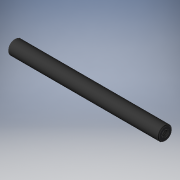
# Autodesk Inventor part: RDOB8-86-WMC4
Saved by Autodesk Inventor 2019 (Build 230136000, 136)
## iProperties
Created: 2022-12-28
Part Number: RDOB8-86-WMC4
Material: Generic
Catalog Web Link: www.cadenas.de
Description: RDOC, RDOB, RDOM, RDSS, RDSSB, RDSSM, RD435S-Rods - Material 1045 Carbon Steel, 1018 Carbon Steel, 4137 Alloy Steel - Outer Diameter Selectable Type
Vendor: MISUMI
Document SubType Name: Modeling
Designer: psAdmin
Manufacturer: MISUMI
Mass: 4.16076 g
Surface Area: 24.2921 cm^2
Volume: 4.16076 cm^3
Density: 1 g/cm^3
Appearance: PSOLRGB-175-175-175
Category: PARTsolutions
Company: MISUMI
Title: RDOB8-86-WMC4
Author: Cadenas PARTsolutions
Comments: Rods - Material 1045 Carbon Steel, 1018 Carbon Steel, 4137 Alloy Steel - Outer Diameter Selectable Type
PSOL_IDENT_0: {$CADENAS_DATA/23d-libs/misumi/metric/22_rods_pipes/rdoc.prj},232 {VTYP=3D},{NB=RDOB8-86-WMC4},{LINA=
PSOL_IDENT_1: RDOB8-86-WMC4},{NN=RDOC, RDOB, RDOM, RDSS, RDSSB, RDSSM, RD435S},{DATE=07.06.2021 02:47:19},{GEOMDAT
PSOL_IDENT_2: E=07.10.2015 00:00:37},{VERSION=},{LINEID=50},{WBVAR=MAT,ST,L,ALT1,MC,WMC},{WBNUMERIC=L,MC,WMC}  {NB=
PSOL_IDENT_3: RDOB8-86-WMC4},{LINA=RDOB8-86-WMC4},{KT=DUMMY},{PN=RDOB8-86-WMC4},{TYPE=RDOB},{MAT=1},{ST=2},{STA='1'
PSOL_IDENT_4: ,'-','2','Black Oxide','3','Electroless Nickel Plating'},{D=8},{DTOL=0/-0.1},{L=86},{LTOL=+/-0.3},{L
PSOL_IDENT_5: 1=[10:500/1]},{C=0.5},{ALT1=2},{ALT1A='3','w/o Tapping','1','with MC (One End Tapping)','2','with WM
PSOL_IDENT_6: C (Both Ends Tapping)'},{MC=0},{MCSA=0},{MCS1=3,4},{WMC=4},{WMCSA=3,4},{WMCS1=3,4},{MMAX=4},{P=0.70}
PSOL_IDENT_7: ,{KDM=3.242},{MATA= '1', '1045 Carbon Steel Equivalent', '2', '1018 Carbon Steel' , '3' , 'SCM435' }
NB: RDOB8-86-WMC4
NN: RDOC, RDOB, RDOM, RDSS, RDSSB, RDSSM, RD435S
NT: Rods - Material 1045 Carbon Steel, 1018 Carbon Steel, 4137 Alloy Steel - Outer Diameter Selectable Type
NBSYN: $PN.
LINA: RDOB8-86-WMC4
CATALOG: Misumi
PN: RDOB8-86-WMC4
MAT: 1045 Carbon Steel Equivalent
ST: Black Oxide
D: 8
DTOL: 0/-0.1
L: 86
LTOL: +/-0.3
C: 0.5
ALT1: with WMC (Both Ends Tapping)
MC: 0
WMC: 4
SUPPLIER: MISUMI
ARTICLENO: RDOB8-86-WMC4
BOMINFO: RDOB8-86-WMC4
CREATOR: CADENAS GmbH
Autodesk Inventor part; units mm, degrees
ref_plane "YZ Plane" through (0, 0, 0) normal (1, 0, 0) x (0, 1, 0)
ref_plane "XZ Plane" through (0, 0, 0) normal (0, 1, 0) x (-1, 0, 0)
ref_plane "XY Plane" through (0, 0, 0) normal (0, 0, 1) x (1, 0, 0)
sketch "Sketch_1" plane through (0, 0, 0) normal (0, 0, 1) x (1, 0, 0)
  line L0 (86, 0) -> (0, 0)
  line L1 (0, 0) -> (0, 3.5)
  line L2 (0, 3.5) -> (0.5, 4)
  line L3 (0.5, 4) -> (85.5, 4)
  line L4 (85.5, 4) -> (86, 3.5)
  line L5 (86, 3.5) -> (86, 0)
  line L6 (86, 0) -> (0, 0)
  constraints: 14 end point
revolve "Revolution1" add sketch "Sketch_1" angle 360 about axis through (86, 0, 0) along (1, 0, 0)
sketch "Sketch2" plane through (0, 0, 0) normal (-1, 0, 0) x (0, 0, 1)
  point P0 (0, 0)
hole "Hole1" at (0, 0, 0) direction (1, 0, 0) diameter 3.242 depth 9.0641 tip angle 120 countersink diameter 4 countersink angle 90 thread size "M4x0.7" class "6H" standard "ISO Metric profile"
sketch "Sketch3" plane through (86, 0, 0) normal (1, 0, 0) x (0, 0, -1)
  point P0 (0, 0)
hole "Hole2" at (86, 0, 0) direction (-1, 0, 0) diameter 3.242 depth 9.0241 tip angle 120 countersink diameter 4 countersink angle 90 thread size "M4x0.7" class "6H" standard "ISO Metric profile"
body "Solid1"
